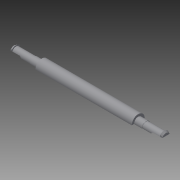
# Autodesk Inventor part: SpoolHandle-axis1
Saved by Autodesk Inventor 2014 (Build 180170000, 170)
## iProperties
Created: 2014-04-04
Part Number: SpoolHandle-axis1
Material: Generic
Document SubType Name: Modeling
Designer: Krzysiek
Density: 1 g/cm^3
Appearance: Default
Author: Krzysiek
Autodesk Inventor part; units mm, degrees
ref_plane "YZ Plane" through (0, 0, 0) normal (1, 0, 0) x (0, 1, 0)
ref_plane "XZ Plane" through (0, 0, 0) normal (0, 1, 0) x (-1, 0, 0)
ref_plane "XY Plane" through (0, 0, 0) normal (0, 0, 1) x (1, 0, 0)
sketch "Sketch1" plane through (0, 0, 0) normal (0, 0, 1) x (1, 0, 0)
  line L0 (43, 5.75) -> (0, 5.75)
  line L1 (0, 5.75) -> (0, 0)
  line L2 (43, 3.75) -> (43, 5.75)
  line L3 (0, 0) -> (67.7321, 0)
  line L4 (43, 3.75) -> (50, 3.75)
  line L5 (50, 3.75) -> (50, 3.5)
  line L6 (50, 3.5) -> (66, 3.5)
  line L7 (67.7321, 0) -> (67.7321, 3.5)
  line L8 (67.7321, 3.5) -> (66, 4.5)
  line L9 (66, 4.5) -> (66, 3.5)
  line L10 (66, 3.5) -> (67.7321, 3.5) construction
  dimension "d5" = 43
  dimension "d6" = 3.5
  dimension "d7" = 3.75
  dimension "d8" = 7
  dimension "d9" = 120
  dimension "d10" = 1
  dimension "d11" = 66
  dimension "d12" = 5.75
  constraints: 22 end point, 3 horizontal, 3 parallel, 3 perpendicular, 2 point on line, 1 collinear
  measures "d5" distance of L0.start L0.end
  measures "d6" distance between parallel lines of L3 L6
  measures "d7" distance between parallel lines of L3 L4
  measures "d8" distance of L2.start L4.end
  measures "d9" angle of L7 L8
  measures "d10" distance of L8.end L6.end
  measures "d11" distance between parallel lines of L9 L1
  measures "d12" distance of L0.end L1.end
revolve "Revolution1" add sketch "Sketch1" angle 180 about axis through (0, 0, 0) along (1, 0, 0)
sketch "Sketch2" plane through (43, 5.75, 0) normal (0, 0, -1) x (-1, 0, 0)
  line L0 (-23, -1.25) -> (-23, -2.25) projected
  line L1 (-24.7321, -2.25) -> (-23, -1.25) projected
  line L2 (-24.7321, -2.25) -> (-24.7321, -9.25) projected
  line L3 (-24.7321, -9.25) -> (-23, -10.25) projected
  line L4 (-23, -10.25) -> (-23, -9.25) projected
  line L5 (-23, -2.25) -> (-15, -2.25)
  line L6 (-15, -2.25) -> (-15, -9.25)
  line L7 (-15, -9.25) -> (-23, -9.25)
  dimension "d14" = 8
  constraints: 6 end point, 2 perpendicular, 1 parallel
  measures "d14" distance of L0.end L5.end
extrude "Extrusion1" cut sketch "Sketch2" against normal blind 1.25
chamfer "Chamfer1" distance 1.25 angle 45 1 edges at (58, 0, 1.25)
sketch "Sketch3" plane through (43, 5.75, 1.25) normal (0, 0, -1) x (-1, 0, 0)
  line L0 (-23, -1.4271) -> (-23, -2.4808) projected
  spline S0 degree 2 poles (-24.7321, -2.4808) (-23.9862, -2.0198) (-23, -1.4271) knots 0 0 0 1 1 1 weights 1 1.008789 1 projected
  spline S1 degree 2 poles (-23, -10.0729) (-23.9862, -9.4802) (-24.7321, -9.0192) knots 0 0 0 1 1 1 weights 1 1.008789 1 projected
  line L1 (-23, -9.0192) -> (-23, -10.0729) projected
  line L2 (-23, -2.4808) -> (-24.7321, -2.4808)
  line L3 (-24.7321, -9.0192) -> (-23, -9.0192)
  point P0 (43, -5.75)
  constraints: 4 end point, 1 parallel, 1 perpendicular, 2 other
extrude "Extrusion2" cut sketch "Sketch3" against normal blind 2
mirror "Mirror1" about plane through (0, 5.75, 0) normal (-1, 0, 0)
body "Solid1"
